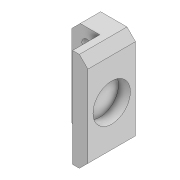
# Autodesk Inventor part: GB-hinge-v1
Saved by Autodesk Inventor 2020 (Build 240168000, 168)
## iProperties
Created: 2021-06-24
Part Number: GB-hinge-v1
Material: Generic
Document SubType Name: Modeling
Designer: Aidan Lee
Density: 1 g/cm^3
Appearance: Default
Author: Aidan Lee
Autodesk Inventor part; units mm, degrees
ref_plane "XZ Plane" through (0, 0, 0) normal (0, 1, 0) x (-1, 0, 0)
ref_plane "XY Plane" through (0, 0, 0) normal (0, 0, 1) x (1, 0, 0)
sketch "Sketch1" plane through (0, 0, 0) normal (0, 0, 1) x (1, 0, 0)
  line L0 (0, 0) -> (140, 0)
  line L1 (140, 0) -> (140, 310)
  line L2 (140, 310) -> (0, 310)
  line L3 (0, 310) -> (0, 0)
  line L4 (15, 295) -> (125, 295) construction
  line L5 (125, 295) -> (125, 15) construction
  line L6 (125, 15) -> (15, 15) construction
  line L7 (15, 15) -> (15, 295) construction
  line L8 (15, 295) -> (125, 295) construction
  line L9 (70, 314.0975) -> (70, 322.6254) construction
  line L10 (15, 295) -> (15, 269.8596) construction
  line L11 (125, 295) -> (125, 292.6022) construction
  line L12 (-24.3067, 155) -> (-34.4998, 155) construction
  line L13 (0, 300.2843) -> (9.7157, 310)
  line L14 (140, 300.2843) -> (130.2843, 310)
  line L15 (0, 9.7157) -> (9.7157, 0)
  line L16 (140, 9.7157) -> (130.2843, 0)
  line L17 (70, 295) -> (70, 310) construction
  line L18 (0, 155) -> (15, 155) construction
  line L19 (23.9173, 286.0827) -> (15, 295) construction
  line L20 (16.5096, 292.7523) -> (17.2477, 293.4904)
  line L21 (23.9173, 286.0827) -> (16.8787, 293.1213) construction
  line L22 (123.4904, 292.7523) -> (122.7523, 293.4904)
  line L23 (15, 17.2679) -> (15, 136.2679) construction
  line L24 (17, 136.2679) -> (17, 17.2679)
  arc A0 (17, 136.2679) -> (15, 136.2679) centre (16, 136.2679) ccw
  arc A1 (14, 16.2679) -> (15, 17.2679) centre (14, 17.2679) ccw construction
  line L25 (14, 16.2679) -> (12, 16.2679) construction
  arc A2 (17, 17.2679) -> (18, 16.2679) centre (18, 17.2679) ccw
  line L26 (20, 16.2679) -> (18, 16.2679)
  line L27 (21, 17.2679) -> (21, 136.2679)
  line L28 (23, 136.2679) -> (23, 17.2679)
  arc A3 (23, 17.2679) -> (24, 16.2679) centre (24, 17.2679) ccw
  arc A4 (23, 136.2679) -> (21, 136.2679) centre (22, 136.2679) ccw
  arc A5 (20, 16.2679) -> (21, 17.2679) centre (20, 17.2679) ccw
  line L29 (26, 16.2679) -> (24, 16.2679)
  line L30 (27, 17.2679) -> (27, 136.2679)
  line L31 (29, 136.2679) -> (29, 17.2679)
  arc A6 (29, 17.2679) -> (30, 16.2679) centre (30, 17.2679) ccw
  arc A7 (29, 136.2679) -> (27, 136.2679) centre (28, 136.2679) ccw
  arc A8 (26, 16.2679) -> (27, 17.2679) centre (26, 17.2679) ccw
  line L32 (32, 16.2679) -> (30, 16.2679)
  line L33 (33, 17.2679) -> (33, 136.2679)
  line L34 (35, 136.2679) -> (35, 17.2679)
  arc A9 (35, 17.2679) -> (36, 16.2679) centre (36, 17.2679) ccw
  arc A10 (35, 136.2679) -> (33, 136.2679) centre (34, 136.2679) ccw
  arc A11 (32, 16.2679) -> (33, 17.2679) centre (32, 17.2679) ccw
  line L35 (38, 16.2679) -> (36, 16.2679)
  line L36 (39, 17.2679) -> (39, 136.2679)
  line L37 (41, 136.2679) -> (41, 17.2679)
  arc A12 (41, 17.2679) -> (42, 16.2679) centre (42, 17.2679) ccw
  arc A13 (41, 136.2679) -> (39, 136.2679) centre (40, 136.2679) ccw
  arc A14 (38, 16.2679) -> (39, 17.2679) centre (38, 17.2679) ccw
  line L38 (44, 16.2679) -> (42, 16.2679)
  line L39 (45, 17.2679) -> (45, 136.2679)
  line L40 (47, 136.2679) -> (47, 17.2679)
  arc A15 (47, 17.2679) -> (48, 16.2679) centre (48, 17.2679) ccw
  arc A16 (47, 136.2679) -> (45, 136.2679) centre (46, 136.2679) ccw
  arc A17 (44, 16.2679) -> (45, 17.2679) centre (44, 17.2679) ccw
  line L41 (50, 16.2679) -> (48, 16.2679)
  line L42 (51, 17.2679) -> (51, 136.2679)
  line L43 (53, 136.2679) -> (53, 17.2679)
  arc A18 (53, 17.2679) -> (54, 16.2679) centre (54, 17.2679) ccw
  arc A19 (53, 136.2679) -> (51, 136.2679) centre (52, 136.2679) ccw
  arc A20 (50, 16.2679) -> (51, 17.2679) centre (50, 17.2679) ccw
  line L44 (56, 16.2679) -> (54, 16.2679)
  line L45 (57, 17.2679) -> (57, 136.2679)
  line L46 (59, 136.2679) -> (59, 17.2679)
  arc A21 (59, 17.2679) -> (60, 16.2679) centre (60, 17.2679) ccw
  arc A22 (59, 136.2679) -> (57, 136.2679) centre (58, 136.2679) ccw
  arc A23 (56, 16.2679) -> (57, 17.2679) centre (56, 17.2679) ccw
  line L47 (62, 16.2679) -> (60, 16.2679)
  line L48 (63, 17.2679) -> (63, 136.2679)
  line L49 (65, 136.2679) -> (65, 17.2679)
  arc A24 (65, 17.2679) -> (66, 16.2679) centre (66, 17.2679) ccw
  arc A25 (65, 136.2679) -> (63, 136.2679) centre (64, 136.2679) ccw
  arc A26 (62, 16.2679) -> (63, 17.2679) centre (62, 17.2679) ccw
  line L50 (68, 16.2679) -> (66, 16.2679)
  line L51 (69, 17.2679) -> (69, 136.2679)
  line L52 (71, 136.2679) -> (71, 17.2679)
  arc A27 (71, 17.2679) -> (72, 16.2679) centre (72, 17.2679) ccw
  arc A28 (71, 136.2679) -> (69, 136.2679) centre (70, 136.2679) ccw
  arc A29 (68, 16.2679) -> (69, 17.2679) centre (68, 17.2679) ccw
  line L53 (74, 16.2679) -> (72, 16.2679)
  line L54 (75, 17.2679) -> (75, 136.2679)
  line L55 (77, 136.2679) -> (77, 17.2679)
  arc A30 (77, 17.2679) -> (78, 16.2679) centre (78, 17.2679) ccw
  arc A31 (77, 136.2679) -> (75, 136.2679) centre (76, 136.2679) ccw
  arc A32 (74, 16.2679) -> (75, 17.2679) centre (74, 17.2679) ccw
  line L56 (80, 16.2679) -> (78, 16.2679)
  line L57 (81, 17.2679) -> (81, 136.2679)
  line L58 (83, 136.2679) -> (83, 17.2679)
  arc A33 (83, 17.2679) -> (84, 16.2679) centre (84, 17.2679) ccw
  arc A34 (83, 136.2679) -> (81, 136.2679) centre (82, 136.2679) ccw
  arc A35 (80, 16.2679) -> (81, 17.2679) centre (80, 17.2679) ccw
  line L59 (86, 16.2679) -> (84, 16.2679)
  line L60 (87, 17.2679) -> (87, 136.2679)
  line L61 (89, 136.2679) -> (89, 17.2679)
  arc A36 (89, 17.2679) -> (90, 16.2679) centre (90, 17.2679) ccw
  arc A37 (89, 136.2679) -> (87, 136.2679) centre (88, 136.2679) ccw
  arc A38 (86, 16.2679) -> (87, 17.2679) centre (86, 17.2679) ccw
  line L62 (92, 16.2679) -> (90, 16.2679)
  line L63 (93, 17.2679) -> (93, 136.2679)
  line L64 (95, 136.2679) -> (95, 17.2679)
  arc A39 (95, 17.2679) -> (96, 16.2679) centre (96, 17.2679) ccw
  arc A40 (95, 136.2679) -> (93, 136.2679) centre (94, 136.2679) ccw
  arc A41 (92, 16.2679) -> (93, 17.2679) centre (92, 17.2679) ccw
  line L65 (98, 16.2679) -> (96, 16.2679)
  line L66 (99, 17.2679) -> (99, 136.2679)
  line L67 (101, 136.2679) -> (101, 17.2679)
  arc A42 (101, 17.2679) -> (102, 16.2679) centre (102, 17.2679) ccw
  arc A43 (101, 136.2679) -> (99, 136.2679) centre (100, 136.2679) ccw
  arc A44 (98, 16.2679) -> (99, 17.2679) centre (98, 17.2679) ccw
  line L68 (104, 16.2679) -> (102, 16.2679)
  line L69 (105, 17.2679) -> (105, 136.2679)
  line L70 (107, 136.2679) -> (107, 17.2679)
  arc A45 (107, 17.2679) -> (108, 16.2679) centre (108, 17.2679) ccw
  arc A46 (107, 136.2679) -> (105, 136.2679) centre (106, 136.2679) ccw
  arc A47 (104, 16.2679) -> (105, 17.2679) centre (104, 17.2679) ccw
  line L71 (110, 16.2679) -> (108, 16.2679)
  line L72 (111, 17.2679) -> (111, 136.2679)
  line L73 (113, 136.2679) -> (113, 17.2679)
  arc A48 (113, 17.2679) -> (114, 16.2679) centre (114, 17.2679) ccw
  arc A49 (113, 136.2679) -> (111, 136.2679) centre (112, 136.2679) ccw
  arc A50 (110, 16.2679) -> (111, 17.2679) centre (110, 17.2679) ccw
  line L74 (116, 16.2679) -> (114, 16.2679)
  line L75 (117, 17.2679) -> (117, 136.2679)
  line L76 (119, 136.2679) -> (119, 17.2679)
  arc A51 (119, 17.2679) -> (120, 16.2679) centre (120, 17.2679) ccw
  arc A52 (119, 136.2679) -> (117, 136.2679) centre (118, 136.2679) ccw
  arc A53 (116, 16.2679) -> (117, 17.2679) centre (116, 17.2679) ccw
  line L77 (122, 16.2679) -> (120, 16.2679)
  line L78 (123, 17.2679) -> (123, 136.2679)
  line L79 (125, 136.2679) -> (125, 17.2679) construction
  arc A54 (125, 17.2679) -> (126, 16.2679) centre (126, 17.2679) ccw construction
  arc A55 (125, 136.2679) -> (123, 136.2679) centre (124, 136.2679) ccw
  arc A56 (122, 16.2679) -> (123, 17.2679) centre (122, 17.2679) ccw
  spline S0 degree 4 poles (16.5096, 292.7523) (14.6512, 290.8939) (16.6332, 288.5857) (14.1324, 255.5259) (27.5104, 252.1329) (46.2634, 240.1563) (54.7125, 235.9841) (66.7216, 222.7724) (65.5, 220.3363) (65.5, 218.384) knots 0 0 0 0 0 0.204369 0.361344 0.535946 0.694753 0.83232 1 1 1 1 1
  line L80 (65.5, 218.384) -> (65.5, 202.0117) construction
  line L81 (74.5, 218.384) -> (74.5, 202.0117) construction
  spline S1 degree 4 poles (123.4904, 292.7523) (125.3488, 290.8939) (123.3668, 288.5857) (125.8676, 255.5259) (112.4896, 252.1329) (93.7366, 240.1563) (85.2875, 235.9841) (73.2784, 222.7724) (74.5, 220.3363) (74.5, 218.384) knots 0 0 0 0 0 0.204369 0.361344 0.535946 0.694753 0.83232 1 1 1 1 1
  line L82 (65.5, 218.384) -> (74.5, 218.384) construction
  line L83 (65.5389, 141.7679) -> (74.4611, 141.7679) construction
  line L84 (70, 141.7679) -> (70, 218.384) construction
  line L85 (70, 218.384) -> (70, 295) construction
  line L86 (65.5, 218.384) -> (15, 218.384) construction
  line L87 (62.8707, 226.1769) -> (62.8707, 218.384) construction
  line L88 (57.0465, 232.5428) -> (57.0465, 218.384) construction
  line L89 (46, 240.6096) -> (46, 218.384) construction
  line L90 (29, 250.3296) -> (29, 218.384) construction
  line L91 (18, 261.7679) -> (18, 218.384) construction
  line L92 (15.4781, 289.1037) -> (15.4781, 218.384) construction
  spline S2 degree 4 poles (65.5, 218.384) (65.5, 215.0405) (62.848, 209.2957) (57.3611, 204.0625) (44.7836, 194.6245) (24.1609, 184.7814) (14.4252, 176.5299) (15, 157.5503) (15, 148.5289) knots 0 0 0 0 0 0.19694 0.347855 0.51086 0.697962 1 1 1 1 1
  line L93 (62.8707, 218.384) -> (62.8707, 210.5911) construction
  line L94 (57.0465, 218.384) -> (57.0465, 204.2251) construction
  line L95 (46, 218.384) -> (46, 196.1584) construction
  line L96 (29, 218.384) -> (29, 186.4384) construction
  line L97 (18, 218.384) -> (18, 175) construction
  spline S3 degree 4 poles (74.5, 218.384) (74.5, 215.0405) (77.152, 209.2957) (82.6389, 204.0625) (95.2164, 194.6245) (115.8391, 184.7814) (125.5748, 176.5299) (125, 157.5503) (125, 148.5289) knots 0 0 0 0 0 0.19694 0.347855 0.51086 0.697962 1 1 1 1 1
  line L98 (125, 148.5289) -> (125, 140.8711) construction
  circle A57 centre (70, 198.7679) radius 1
  circle A58 centre (70, 184.7679) radius 1
  circle A59 centre (70, 170.7679) radius 1
  circle A60 centre (70, 156.7679) radius 1
  circle A61 centre (70, 142.7679) radius 1
  line L99 (-110.1015, 148.4668) -> (-137.337, 121.2312) construction
  line L100 (-137.337, 121.2312) -> (-99.9418, 121.2312) construction
  circle A62 centre (63, 191.7679) radius 1
  line L101 (-29.4032, 198.7679) -> (-29.4032, 184.7679) construction
  line L102 (63, 191.7679) -> (70, 198.7679) construction
  circle A63 centre (63, 177.7679) radius 1
  circle A64 centre (63, 163.7679) radius 1
  circle A65 centre (63, 149.7679) radius 1
  line L103 (70, 184.7679) -> (70, 170.7679) construction
  line L104 (70, 170.7679) -> (70, 156.7679) construction
  line L105 (70, 156.7679) -> (70, 142.7679) construction
  line L106 (63, 191.7679) -> (56, 184.7679) construction
  line L107 (56, 184.7679) -> (49, 177.7679) construction
  line L108 (49, 177.7679) -> (42, 170.7679) construction
  line L109 (42, 170.7679) -> (35, 163.7679) construction
  line L110 (35, 163.7679) -> (28, 156.7679) construction
  line L111 (28, 156.7679) -> (21, 149.7679) construction
  line L112 (21, 149.7679) -> (14, 142.7679) construction
  line L113 (14, 156.7679) -> (21, 163.7679) construction
  line L114 (21, 163.7679) -> (28, 170.7679) construction
  line L115 (28, 170.7679) -> (35.279, 178.047) construction
  line L116 (35.279, 178.047) -> (42, 184.7679) construction
  circle A66 centre (56, 184.7679) radius 1
  circle A67 centre (49, 177.7679) radius 1
  circle A68 centre (42, 184.7679) radius 1
  circle A69 centre (42, 170.7679) radius 1
  circle A70 centre (35, 177.7679) radius 1
  circle A71 centre (28, 170.7679) radius 1
  circle A72 centre (35, 163.7679) radius 1
  circle A73 centre (49, 163.7679) radius 1
  circle A74 centre (56, 170.7679) radius 1
  circle A75 centre (21, 163.7679) radius 1
  circle A76 centre (21, 149.7679) radius 1
  circle A77 centre (49, 191.7679) radius 1
  circle A78 centre (42, 156.7679) radius 1
  circle A79 centre (28, 156.7679) radius 1
  circle A80 centre (28, 142.7679) radius 1
  circle A81 centre (35, 149.7679) radius 1
  circle A82 centre (42, 142.7679) radius 1
  circle A83 centre (49, 149.7679) radius 1
  circle A84 centre (56, 156.7679) radius 1
  circle A85 centre (56, 142.7679) radius 1
  circle A86 centre (77, 191.7679) radius 1
  circle A87 centre (77, 177.7679) radius 1
  circle A88 centre (77, 163.7679) radius 1
  circle A89 centre (77, 149.7679) radius 1
  circle A90 centre (84, 184.7679) radius 1
  circle A91 centre (91, 177.7679) radius 1
  circle A92 centre (98, 184.7679) radius 1
  circle A93 centre (98, 170.7679) radius 1
  circle A94 centre (105, 177.7679) radius 1
  circle A95 centre (112, 170.7679) radius 1
  circle A96 centre (105, 163.7679) radius 1
  circle A97 centre (91, 163.7679) radius 1
  circle A98 centre (84, 170.7679) radius 1
  circle A99 centre (119, 163.7679) radius 1
  circle A100 centre (119, 149.7679) radius 1
  circle A101 centre (91, 191.7679) radius 1
  circle A102 centre (98, 156.7679) radius 1
  circle A103 centre (112, 156.7679) radius 1
  circle A104 centre (112, 142.7679) radius 1
  circle A105 centre (105, 149.7679) radius 1
  circle A106 centre (98, 142.7679) radius 1
  circle A107 centre (91, 149.7679) radius 1
  circle A108 centre (84, 156.7679) radius 1
  circle A109 centre (84, 142.7679) radius 1
  line L117 (15, 148.5289) -> (15, 140.2675)
  line L118 (125, 148.5289) -> (125, 140.2675)
  spline S4 degree 4 poles (17.2477, 293.4904) (18.1955, 294.4381) (19.6714, 295.0826) (20.7017, 295) (21.8623, 295) knots 0 0 0 0 0 1 1 1 1 1
  spline S5 degree 3 poles (122.7523, 293.4904) (121.4886, 294.7541) (119.4432, 295.1927) (118.1377, 295) knots 0 0 0 0 1 1 1 1
  line L119 (118.1377, 295) -> (21.8623, 295)
  line L120 (16.8787, 293.1213) -> (23.2316, 286.7684) construction
  arc A110 (19, 310) -> (0, 291) centre (19, 291) ccw construction
  arc A111 (19, 295) -> (15, 291) centre (19, 291) ccw construction
  line L121 (19, 291) -> (10, 291) construction
  line L122 (19, 291) -> (19, 300) construction
  line L123 (16.1716, 293.8284) -> (5.565, 304.435) construction
  circle A112 centre (10.8683, 299.1317) radius 2
  line L124 (9.8231, 300.915) -> (9.085, 300.1769) construction
  line L125 (11.9134, 297.3485) -> (12.6515, 298.0866) construction
  circle A113 centre (70, 302.5) radius 2
  circle A114 centre (7.5, 155) radius 2
  circle A115 centre (7.5, 227.0659) radius 2
  line L126 (7.5, 155) -> (7.5, 227.0659) construction
  line L127 (7.5, 227.0659) -> (7.5, 299.1317) construction
  arc A116 (140, 291) -> (121, 310) centre (121, 291) ccw construction
  arc A117 (125, 291) -> (121, 295) centre (121, 291) ccw construction
  circle A118 centre (129.1317, 299.1317) radius 2
  circle A119 centre (132.5, 155) radius 2
  circle A120 centre (132.5, 227.0659) radius 2
  circle A121 centre (10.8683, 10.8683) radius 2
  circle A122 centre (70, 7.5) radius 2
  circle A123 centre (7.5, 82.9341) radius 2
  circle A124 centre (132.5, 82.9341) radius 2
  circle A125 centre (129.1317, 10.8683) radius 2
  arc A126 (0, 19) -> (19, 0) centre (19, 19) ccw construction
  arc A127 (15, 19) -> (19, 15) centre (19, 19) ccw construction
  arc A128 (121, 0) -> (140, 19) centre (121, 19) ccw construction
  arc A129 (121, 15) -> (125, 19) centre (121, 19) ccw construction
  circle A130 centre (10.8683, 299.1317) radius 7.5 construction
  line L128 (4.4716, 303.3416) -> (6.8718, 305.7419) construction
  line L129 (15, 140.2675) -> (15, 136.2679)
  line L130 (125, 140.2675) -> (125, 136.2679)
  line L131 (140, -47.2692) -> (140, -78.7692) construction
  line L132 (280, 310) -> (280, 0)
  circle A131 centre (272.5, 155) radius 2
  line L133 (282, 166) -> (289, 166) construction
  line L134 (289, 166) -> (289, 144) construction
  line L135 (289, 144) -> (282, 144) construction
  line L136 (282, 144) -> (282, 166) construction
  line L137 (280, 184) -> (282, 184)
  line L138 (282, 184) -> (282, 178.7679) construction
  line L139 (289, 166) -> (289, 168)
  circle A132 centre (272.5, 175) radius 3
  line L140 (263.5, 175) -> (263.5, 155)
  arc A133 (272.5, 184) -> (263.5, 175) centre (272.5, 175) ccw
  line L141 (280, 184) -> (272.5, 184)
  line L142 (263.5, 166) -> (280, 184) construction
  point P0 (70, 318.3615)
  point P1 (-29.4032, 155)
  point P2 (65.2876, 221.8871)
  point P3 (122, 261.7679)
  point P4 (111, 250.3296)
  point P5 (94, 240.6096)
  point P6 (82.9535, 232.5428)
  point P7 (74.7124, 221.8871)
  point P8 (124.5219, 289.1037)
  point P9 (77.1293, 210.5911)
  point P10 (82.9535, 204.2251)
  point P11 (94, 196.1584)
  point P12 (111, 186.4384)
  point P13 (122, 175)
  point P14 (-29.4032, 191.7679)
  point P15 (70, 177.7679)
  point P16 (70, 163.7679)
  point P17 (70, 149.7679)
  point P18 (19.6961, 294.835)
  point P19 (120.3039, 294.835)
  point P20 (9.4541, 300.5459)
  point P21 (12.2825, 297.7175)
  point P22 (140, -63.0192)
  point P23 (140, 155)
  point P24 (289, 155)
  point P25 (271.75, 175)
  dimension "d163" = 4
  dimension "d0" = 140
  dimension "d1" = 310
  dimension "d2" = 15
  dimension "d114" = 135
  dimension "d124" = 2
  dimension "d126" = 1
  dimension "d128" = 2
  dimension "d136" = 6
  dimension "d141" = 9
  dimension "d142" = 5.5
  dimension "pegd" = 2
  dimension "d147" = 14
  dimension "d152" = 45
  dimension "d158" = 45
  dimension "d161" = 4
  dimension "d164" = 5.5
  dimension "d168" = 15
  dimension "d169" = 1
  dimension "d170" = 1
  dimension "d171" = 1
  dimension "d172" = 120
  dimension "d175" = 7
  dimension "d176" = 22
  dimension "d177" = 2
  dimension "d178" = 6
  dimension "d179" = 18
  dimension "d212" = 16.5
  constraints: 286 end point, 153 point on circle, 133 centre point, 73 symmetric about line, 46 point on line, 35 horizontal alignment, 27 vertical alignment, 25 equal radius, 23 midpoint, 21 vertical, 16 equal length, 14 horizontal, 14 parallel, 14 perpendicular, 13 coincident, 12 collinear, 9 tangent, 401 other
  measures "d0" distance of L0.start L0.end
  measures "d1" distance of L2.end L0.start
  measures "d2" distance between parallel lines of L2 L4
  measures "d114" angle of L3 L13
  measures "d124" distance between parallel lines of L23 L24
  measures "d126" radius of A1
  measures "d128" distance of L25.start L25.end
  measures "d136" distance of L25.start L26.start
  measures "d141" distance between parallel lines of L81 L80
  measures "d142" distance from line of A28.centre L83
  measures "pegd" diameter of A57
  measures "d147" distance of L102.end L103.start
  measures "d152" angle of L100 L99
  measures "d158" angle of L4 L21
  measures "d161" radius of A111
  measures "d164" distance edge to line of A110 L124
  measures "d168" diameter of A130
  measures "d169" distance between parallel lines of L13 L128
  measures "d170" distance from line of L123.start L20
  measures "d171" horizontal distance between centres of A127 A2
  measures "d172" distance from line of L26 A0.centre
  measures "d175" distance of L134.end L135.end
  measures "d176" distance of L133.end L134.end
  measures "d177" distance between parallel lines of L132 L136
  measures "d178" diameter of A132
  measures "d179" distance between parallel lines of L137 L133
  measures "d212" distance between parallel lines of L132 L140
ref_plane "Work Plane2" through (280, 310, 0) normal (1, 0, 0) x (0, -1, 0)
sketch "Sketch3" plane through (280, 310, 0) normal (1, 0, 0) x (0, -1, 0)
  line L0 (223.8854, -8) -> (118.8331, -8) construction
  line L1 (118.8331, -8) -> (118.8331, 8) construction
  line L2 (118.8331, 8) -> (223.8854, 8)
  line L3 (223.8854, 8) -> (223.8854, -8) construction
  circle A0 centre (155, 6) radius 11
  circle A1 centre (155, 6) radius 14 construction
  line L4 (126, -8) -> (184, -8)
  line L5 (184, -8) -> (184, 20)
  line L6 (184, 20) -> (126, 20)
  line L7 (126, 20) -> (126, -8)
  line L8 (126, 18) -> (184, 18)
  line L9 (151.9614, 17) -> (158.9718, 17) construction
  point P0 (310, 0)
  point P1 (155, 0)
  point P2 (126, 0)
  point P3 (126, 0)
  point P4 (126, 0)
  point P5 (126, 0)
  point P6 (118.8331, 0)
  point P7 (155, 20)
  point P8 (126, 8)
  point P9 (184, 8)
  dimension "d189" = 28
  dimension "thickness" = 16
  dimension "d188" = 22
  dimension "d191" = 1
  constraints: 20 end point, 5 parallel, 4 horizontal, 4 point on line, 3 vertical alignment, 2 coincident, 2 midpoint, 2 perpendicular, 1 centre point, 1 horizontal alignment, 1 tangent, 2 other
  measures "thickness" distance of L0.end L1.end
  measures "d188" diameter of A0
  measures "d191" distance between parallel lines of L8 L9
extrude "Extrusion2" add sketch "Sketch3" along normal blind 2 contours A0 L2 | L2 A0
extrude "Extrusion3" add sketch "Sketch3" along normal up to surface (9 mm away) contours L7 L8 L5 L2 A0 | L2 A0 L5 L4 L7 | L7 L6 L5 L8
extrude "Extrusion4" add sketch "Sketch3" against normal up to surface (16.5 mm away) contours L7 L8 L5 L2 A0 | A0 L2 | L7 L6 L5 L8 picked at (157.7729, 12.5)
sketch "Sketch4" plane through (289, 126, -20) normal (0, 0, -1) x (-1, 0, 0)
  circle A0 centre (16.5, 49) radius 3 projected
  line L0 (313.3067, 29) -> (323.4998, 29) construction
  line L1 (9, 29) -> (-7.0831, 29)
  circle A1 centre (16.5, 9) radius 3
  point P0 (289, -126)
  constraints: 2 end point, 2 symmetric about line, 1 centre point, 1 horizontal, 1 other
hole "Hole1" at (272.5, 175, -20) at (272.5, 135, -20) direction (0, 0, 1) diameter 6 end through all countersink diameter 13.44 countersink angle 90
chamfer "Chamfer1" distance 5 angle 45 2 edges at (289, 184, -6) (289, 126, -6)
chamfer "Chamfer2" distance 5 angle 45 2 edges at (263.5, 184, -14) (263.5, 126, -14)
body "Solid2"
